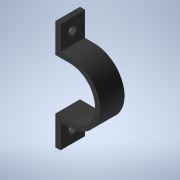
# Autodesk Inventor part: 12_Motor_Fixation
Saved by Autodesk Inventor 2021 (Build 250183000, 183)
## iProperties
Created: 2021-08-05
Part Number: 12_Motor_Fixation
Material: Generisch
Document SubType Name: Modeling
Designer: User
Density: 1 g/cm^3
Appearance: Vorgabe
Author: User
## iProperties of the stored document _3D-Druck.ipt
Created: 2021-08-05
Part Number: _3D-Druck
Material: Generisch
Document SubType Name: Modeling
Designer: User
Density: 1 g/cm^3
Appearance: Vorgabe
Author: User
Autodesk Inventor part; units mm, degrees
ref_plane "YZ Plane" through (0, 0, 0) normal (1, 0, 0) x (0, 1, 0)
ref_plane "XZ Plane" through (0, 0, 0) normal (0, 1, 0) x (-1, 0, 0)
ref_plane "XY Plane" through (0, 0, 0) normal (0, 0, 1) x (1, 0, 0)
sketch "Skizze1" plane through (0, 0, 0) normal (0, 0, 1) x (1, 0, 0)
  arc A0 (-12.4981, -6.2168) -> (-0.2168, 6.4981) centre (0, -6) ccw projected
  arc A1 (-0.2168, 6.4981) -> (-12.4981, -6.2168) centre (0, -6) ccw projected
  line L0 (-12.4401, -116.2323) -> (-16.2556, 103.7346) projected
  line L1 (-6.95, -18.5) -> (0, -18.5)
  arc A2 (0, -18.5) -> (0, 6.5) centre (0, -6) ccw
  line L2 (0, 6.5) -> (-6.95, 6.5)
  line L3 (-6.95, 6.5) -> (-6.95, 20.9)
  line L4 (-6.95, 20.9) -> (-4.55, 20.9)
  line L5 (-4.55, 20.9) -> (-4.55, 8.9)
  line L6 (-4.55, 8.9) -> (0, 8.9)
  arc A3 (0, -20.9) -> (0, 8.9) centre (0, -6) ccw
  line L7 (0, -20.9) -> (-4.55, -20.9)
  line L8 (-4.55, -20.9) -> (-4.55, -32.9)
  line L9 (-4.55, -32.9) -> (-6.95, -32.9)
  line L10 (-6.95, -32.9) -> (-6.95, -18.5)
  point P0 (0, 0)
  point P1 (-14.35, 20.9)
  point P2 (-14.35, 6.5)
  point P3 (0, 6.5)
  point P4 (0, -18.5)
  point P5 (-14.35, -18.5)
  point P6 (-14.35, -32.9)
  dimension "d0" = 2.4
  dimension "d1" = 2.4
  dimension "d2" = 2.4
  dimension "d4" = 12.5
  dimension "d5" = 7.4
  dimension "d7" = 12.5
  dimension "d8" = 12
  constraints: 20 end point, 5 perpendicular, 4 parallel, 4 point on circle, 3 collinear, 3 tangent, 2 centre point, 2 concentric, 1 vertical
  measures "d0" distance between parallel lines of L10 L8
  measures "d1" distance between parallel lines of L1 L7
  measures "d2" radial gap between concentric circles of A2 A3
  measures "d4" radius of A1
  measures "d7" radius of A2
  measures "d8" distance of L4.end L5.end
extrude "Extrusion1" add sketch "Skizze1" against normal blind 12 contours A0 L2 L3 L4 L5 L6 A3 L7 L8 L9 L10 L1
sketch "Skizze2" plane through (-4.55, 8.9, 0) normal (1, 0, 0) x (0, 0, -1)
  line L0 (0, 0) -> (12, 0) projected
  line L1 (12, -2.4) -> (12, 12) projected
  line L2 (0, 0) -> (12, 12) construction
  circle A0 centre (6, 6) radius 2
  line L3 (12, -41.8) -> (12, -27.4) construction
  line L4 (12, -41.8) -> (0, -29.8) construction
  line L5 (0, -27.4) -> (0, -41.8) construction
  circle A1 centre (6, -35.8) radius 2
  point P0 (0, -8.9)
  dimension "d11" = 4
  constraints: 4 end point, 2 centre point, 2 midpoint, 1 equal radius
  measures "d11" diameter of A0
extrude "Extrusion2" cut sketch "Skizze2" against normal through all
equation "\"d1\" = d0"
equation "\"d2\" = d0"
equation "\"d7\" = d4"
equation "\"d9\" = d8"
